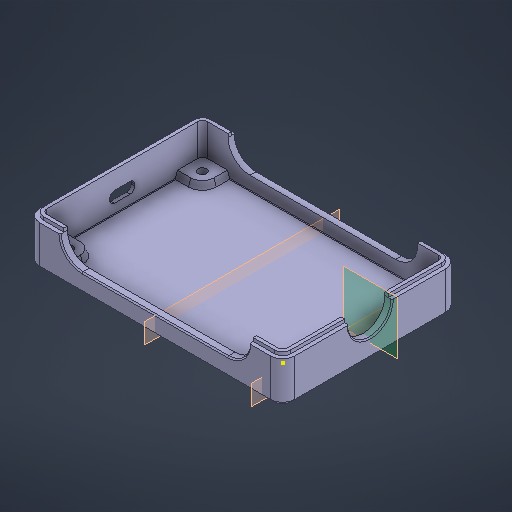
# Autodesk Inventor part: case1
Saved by Autodesk Inventor 2025.2 (Build 292293000, 293)
## iProperties
Created: 2025-10-04
Part Number: case1
Material: Generic
Document SubType Name: Modeling
Designer: micyg
Density: 1 g/cm^3
Appearance: Default
Author: micyg
## iProperties of the stored document case1_3DPrint.ipt
Created: 2025-10-05
Part Number: case1_3DPrint
Material: Generic
Document SubType Name: Modeling
Designer: micyg
Density: 1 g/cm^3
Appearance: Default
Author: micyg
Autodesk Inventor part; units mm, degrees
ref_plane "YZ Plane" through (0, 0, 0) normal (1, 0, 0) x (0, 1, 0)
ref_plane "XZ Plane" through (0, 0, 0) normal (0, 1, 0) x (-1, 0, 0)
ref_plane "XY Plane" through (0, 0, 0) normal (0, 0, 1) x (1, 0, 0)
sketch "Sketch1" plane through (0, 0, 0) normal (0, 1, 0) x (-1, 0, 0)
  line L0 (0, 0) -> (105.2, 0)
  line L1 (105.2, 0) -> (105.2, -72.2)
  line L2 (105.2, -72.2) -> (0, -72.2)
  line L3 (0, -72.2) -> (0, 0)
  line L4 (0, -72.2) -> (105.2, 0) construction
  line L5 (3.6, -3.6) -> (101.6, -3.6) construction
  line L6 (101.6, -3.6) -> (101.6, -68.6) construction
  line L7 (101.6, -68.6) -> (3.6, -68.6) construction
  line L8 (3.6, -68.6) -> (3.6, -3.6) construction
  line L9 (3.6, -3.6) -> (101.6, -68.6) construction
  line L10 (101.6, -3.6) -> (3.6, -68.6) construction
  point P0 (52.6, -36.1)
  dimension "d17" = 98
  dimension "d18" = 65
  dimension "d21" = 72.2
  dimension "d22" = 105.2
  constraints: 22 end point, 4 parallel, 3 midpoint, 2 horizontal, 2 perpendicular
  measures "d17" distance of L6.end L7.end
  measures "d18" distance of L5.end L6.end
  measures "d21" distance between parallel lines of L2 L0
  measures "d22" distance between parallel lines of L3 L1
extrude "Extrusion1" add sketch "Sketch1" along normal blind 17.5
ref_plane "Work Plane7" through (0, 17.5, -36.1) normal (0, 0, -1) x (-1, 0, 0)
fillet "Fillet3" radius 5 4 edges at (-105.2, 8.75, -72.2) (-105.2, 8.75, 0) (0, 8.75, -72.2) (0, 8.75, 0)
chamfer "Chamfer1" distance 2 angle 45 8 edges at (0, 0, -36.1) (-1.4645, 0, -70.7355) (-52.6, 0, -72.2) (-103.7355, 0, -70.7355) (-105.2, 0, -36.1) (-103.7355, 0, -1.4645) (-52.6, 0, 0) (-1.4645, 0, -1.4645)
shell "Shell2" thickness 3 removed faces 1 at (-36.7333, 17.5, -48.1333)
sketch "Sketch2" plane through (-100.2, 3, -69.2) normal (0, 1, 0) x (1, 0, 0)
  line L0 (91.5, -5.6) -> (3.5, -5.6) construction
  line L1 (3.5, -5.6) -> (3.5, -60.6) construction
  line L2 (3.5, -60.6) -> (91.5, -60.6) construction
  line L3 (91.5, -60.6) -> (91.5, -5.6) construction
  arc A0 (91.5, -55.85) -> (86.75, -60.6) centre (91.5, -60.6) ccw
  line L4 (95, 0) -> (0, 0) construction
  arc A1 (-2, -64.2) -> (0, -66.2) centre (0, -64.2) ccw projected
  line L5 (-2, -64.2) -> (-2, -2) projected
  arc A2 (0, 0) -> (-2, -2) centre (0, -2) ccw projected
  line L6 (0, 0) -> (95.2, 0) projected
  arc A3 (97.2, -2) -> (95.2, 0) centre (95.2, -2) ccw projected
  line L7 (97.2, -2) -> (97.2, -64.2) projected
  arc A4 (95.2, -66.2) -> (97.2, -64.2) centre (95.2, -64.2) ccw projected
  line L8 (95.2, -66.2) -> (0, -66.2) projected
  arc A5 (95.2, -69.2) -> (100.2, -64.2) centre (95.2, -64.2) ccw projected
  line L9 (100.2, -64.2) -> (100.2, -2) projected
  arc A6 (100.2, -2) -> (95.2, 3) centre (95.2, -2) ccw projected
  line L10 (95.2, 3) -> (0, 3) projected
  arc A7 (0, 3) -> (-5, -2) centre (0, -2) ccw projected
  line L11 (-5, -2) -> (-5, -64.2) projected
  arc A8 (-5, -64.2) -> (0, -69.2) centre (0, -64.2) ccw projected
  line L12 (0, -69.2) -> (95.2, -69.2) projected
  line L13 (91.5, -55.85) -> (97.2, -55.85)
  line L14 (86.75, -60.6) -> (86.75, -66.2)
  circle A9 centre (91.5, -60.6) radius 1.75
  line L15 (-5, -2) -> (-5, -64.2) projected
  line L16 (-5, -33.1) -> (100.2, -33.1) construction
  line L17 (47.6, -69.2) -> (47.6, 3) construction
  line L18 (3.5, -60.6) -> (91.5, -5.6) construction
  line L19 (47.5, -5.6) -> (47.5, -60.6) construction
  line L20 (-1.5, -0.6) -> (96.5, -0.6) construction
  line L21 (96.5, -0.6) -> (96.5, -65.6) construction
  line L22 (96.5, -65.6) -> (-1.5, -65.6) construction
  line L23 (-1.5, -65.6) -> (-1.5, -0.6) construction
  line L24 (-1.5, -0.6) -> (96.5, -65.6) construction
  arc A10 (86.75, -5.6) -> (91.5, -10.35) centre (91.5, -5.6) ccw
  line L25 (91.5, -10.35) -> (97.2, -10.35)
  line L26 (86.75, -5.6) -> (86.75, 0)
  circle A11 centre (91.5, -5.6) radius 1.75
  arc A12 (8.25, -60.6) -> (3.5, -55.85) centre (3.5, -60.6) ccw
  line L27 (8.25, -60.6) -> (8.25, -66.2)
  circle A13 centre (3.5, -60.6) radius 1.75
  arc A14 (3.5, -10.35) -> (8.25, -5.6) centre (3.5, -5.6) ccw
  line L28 (8.25, -5.6) -> (8.25, 0)
  circle A15 centre (3.5, -5.6) radius 1.75
  line L29 (3.5, -10.35) -> (-2, -10.35)
  line L30 (3.5, -55.85) -> (-2, -55.85)
  point P0 (100.2, -69.2)
  point P1 (47.5, -33.1)
  point P2 (47.5, -33.1)
  point P3 (97.2, -10.35)
  point P4 (8.25, 0)
  dimension "d13" = 88
  dimension "d14" = 55
  dimension "d25" = 3.5
  dimension "d26" = 3
  dimension "d73" = 65
  dimension "d74" = 98
  dimension "d75" = 0.5
  dimension "d76" = 0.7
  constraints: 42 end point, 16 symmetric about line, 9 midpoint, 9 point on circle, 8 centre point, 7 point on line, 4 parallel, 3 coincident, 3 perpendicular, 3 tangent, 2 horizontal, 6 other
  measures "d13" distance between parallel lines of L1 L3
  measures "d14" distance of L2.end L0.start
  measures "d25" diameter of A9
  measures "d26" radial gap between concentric circles of A0 A9
  measures "d73" distance of L20.end L21.end
  measures "d74" distance of L20.start L20.end
  measures "d75" distance between parallel lines of L5 L23
  measures "d76" distance between parallel lines of L21 L7
extrude "Extrusion2" add sketch "Sketch2" along normal blind 2.75 contours L13 L7 A4 L8 L14 A0 | L25 A10 L26 L6 A3 L7 | L8 A1 L5 L30 A12 L27 | L28 A14 L29 L5 A2 L6
ref_plane "Work Plane1" through (-52.6, 17.5, -3) normal (-1, 0, 0) x (0, -1, 0)
ref_plane "Work Plane2" through (-3, 17.5, -36.1) normal (0, 0, 1) x (1, 0, 0)
ref_plane "Work Plane5" through (-52.7, 3, -36.1) normal (1, 0, 0) x (0, 0, -1)
ref_plane "Work Plane6" through (-8.7, 3, -8.6) normal (1, 0, 0) x (0, 0, -1)
sketch "Sketch12" plane through (-8.7, 3, -8.6) normal (1, 0, 0) x (0, 0, -1)
  line L0 (0, 2.75) -> (-5.6, 2.75) projected
  line L1 (-3.6, 2.75) -> (-5.6, 2.75) projected
  line L2 (4.75, 2.75) -> (-3.6, 2.75) projected
  line L3 (4.75, 2.75) -> (0, 2.75) projected
  line L4 (-1.75, 2.75) -> (1.75, 2.75) projected
  line L5 (-1.75, 2.75) -> (1.75, 2.75) projected
  line L6 (1.75, 0) -> (-1.75, 0) projected
  line L7 (-1.75, 2.75) -> (-1.75, 0) projected
  line L8 (1.75, 2.75) -> (1.75, 0) projected
  line L9 (-8.6, 14.5) -> (-8.6, -1) projected
  line L10 (-8.6, -1) -> (-8.6, 14.5) projected
  line L11 (-1.75, 0) -> (-3, -1.25)
  line L12 (-3, -1.25) -> (-3, -3)
  line L13 (-1.75, 0) -> (0, 0)
  line L14 (-1.75, 0) -> (0, 0)
  line L15 (0, 0) -> (0, -3)
  line L16 (1.75, 0) -> (3, -1.25)
  line L17 (3, -1.25) -> (3, -3)
  line L18 (-6.6, -3) -> (-8.6, -1) projected
  line L19 (-8.6, -1) -> (-3.6, -1) projected
  line L20 (-3.6, -3) -> (-3.6, -1) projected
  line L21 (-3.6, -3) -> (-6.6, -3) projected
  line L22 (-3.6, -3) -> (-3.6, -1) projected
  line L23 (-3.6, -1) -> (58.6, -1) projected
  line L24 (58.6, -3) -> (58.6, -1) projected
  line L25 (58.6, -3) -> (-3.6, -3) projected
  line L26 (-8.6, -1) -> (-3.6, -1) projected
  line L27 (-8.6, -1) -> (-8.6, 14.5) projected
  line L28 (-8.6, 14.5) -> (-3.6, 14.5) projected
  line L29 (-3.6, 14.5) -> (-3.6, -1) projected
  point P0 (-8.6, -3)
  dimension "d77" = 45
  dimension "d78" = 6
  constraints: 14 end point, 3 symmetric about line, 2 point on line, 1 collinear, 1 midpoint, 1 perpendicular
  measures "d77" angle of L12 L11
  measures "d78" distance between parallel lines of L17 L12
revolve "Revolution2" cut sketch "Sketch12" angle 360 about axis through (-8.7, 3, -8.6) along (0, -1, 0) contours L16 L23 L15 L6 | L16 L17 L25 L15 L23
mirror "Mirror6" about plane through (-3, 17.5, -36.1) normal (0, 0, 1) of "Revolution2"
mirror "Mirror7" about plane through (-52.7, 3, -36.1) normal (1, 0, 0) of "Revolution2", "Mirror6"
draft "FaceDraft1" angle 20 pull direction (0, 1, 0) faces at (-11.3758, 4.8333, -12.5246) (-13.45, 4.8333, -4.9475) (-4.9809, 4.8333, -13.35) (-13.4367, 3.9167, -63.245) (-4.9809, 4.8333, -58.85) (-13.45, 4.8333, -67.2525) (-92.7754, 4.8333, -11.2758) (-100.2858, 4.8333, -13.35) (-91.95, 4.8333, -4.9475) (-94.9646, 4.8333, -59.1783) (-91.95, 4.8333, -67.2525) (-100.2858, 4.8333, -58.85) fixed edges at (-12.0588, 5.75, -11.9588) (-13.45, 5.75, -5.8) (-5.85, 5.75, -13.35) (-12.0588, 5.75, -60.2412) (-5.85, 5.75, -58.85) (-13.45, 5.75, -66.4) (-93.3412, 5.75, -11.9588) (-99.45, 5.75, -13.35) (-91.95, 5.75, -5.8) (-93.3412, 5.75, -60.2412) (-91.95, 5.75, -66.4) (-99.45, 5.75, -58.85)
sketch "Sketch19" plane through (-5, 17.5, -72.2) normal (0, 0, -1) x (-1, 0, 0)
  line L0 (95.2, -15.5) -> (0, -15.5) construction
  line L1 (95.2, 0) -> (95.2, -15.5) construction
  line L2 (0, 0) -> (95.2, 0) construction
  line L3 (0, -15.5) -> (0, 0) construction
  line L4 (47.7, -21.28) -> (47.7, 5.18) construction
  line L5 (8.7, -9) -> (86.7, -9) construction
  line L6 (86.7, -9) -> (86.7, 9)
  line L7 (86.7, 9) -> (8.7, 9)
  line L8 (8.7, 9) -> (8.7, -9)
  line L9 (8.7, -9) -> (86.7, 9) construction
  line L10 (86.7, -9) -> (8.7, 9) construction
  arc A0 (77.7, -9) -> (77.7, 9) centre (77.7, 0) ccw
  arc A1 (17.7, 9) -> (17.7, -9) centre (17.7, 0) ccw
  line L11 (17.7, -9) -> (77.7, -9)
  line L12 (77.7, 9) -> (17.7, 9)
  point P0 (-5, -17.5)
  point P1 (47.7, 0)
  point P2 (86.7, 0)
  point P3 (8.7, 0)
  point P4 (47.7, 0)
  point P5 (47.7, 0)
  dimension "d103" = 78
  dimension "d104" = 9
  constraints: 16 end point, 8 point on line, 5 tangent, 4 midpoint, 4 point on circle, 2 centre point, 2 horizontal, 2 parallel, 1 perpendicular
  measures "d103" distance between parallel lines of L8 L6
  measures "d104" radius of A0
extrude "Extrusion13" cut sketch "Sketch19" against normal up to surface (3 mm away)
mirror "Mirror9" about plane through (0, 17.5, -36.1) normal (0, 0, -1) of "Extrusion13"
sketch "Sketch20" plane through (0, 17.5, -5) normal (1, 0, 0) x (0, 0, -1)
  line L0 (62.2, -15.5) -> (0, -15.5) construction
  line L1 (62.2, 0) -> (62.2, -15.5) construction
  line L2 (0, 0) -> (62.2, 0) construction
  line L3 (0, -15.5) -> (0, 0) construction
  line L4 (31.1, 3.5) -> (31.1, -21) construction
  circle A0 centre (31.1, 0) radius 9
  point P0 (-5, -17.5)
  dimension "d109" = 18
  constraints: 1 centre point, 1 midpoint, 1 point on line
  measures "d109" diameter of A0
extrude "Extrusion14" cut sketch "Sketch20" against normal up to surface (3 mm away)
sketch "Sketch21" plane through (-105.2, 17.5, -67.2) normal (-1, 0, 0) x (0, 0, 1)
  line L0 (31.1, -9.65) -> (31.1, -9.85) projected
  line L1 (34.29, -9.85) -> (31.1, -9.85) projected
  arc A0 (34.29, -9.85) -> (35.57, -8.57) centre (34.29, -8.57) ccw projected
  line L2 (35.57, -7.97) -> (35.57, -8.57) projected
  arc A1 (35.57, -7.97) -> (34.29, -6.69) centre (34.29, -7.97) ccw projected
  line L3 (31.1, -6.69) -> (34.29, -6.69) projected
  line L4 (31.1, -6.69) -> (31.1, -6.89) projected
  line L5 (31.1, -6.89) -> (34.29, -6.89) projected
  arc A2 (35.37, -7.97) -> (34.29, -6.89) centre (34.29, -7.97) ccw projected
  line L6 (35.37, -7.97) -> (35.37, -8.57) projected
  arc A3 (34.29, -9.65) -> (35.37, -8.57) centre (34.29, -8.57) ccw projected
  line L7 (34.29, -9.65) -> (31.1, -9.65) projected
  line L8 (31.1, -9.65) -> (31.1, -9.85) projected
  line L9 (27.91, -9.65) -> (31.1, -9.65) projected
  arc A4 (26.83, -8.57) -> (27.91, -9.65) centre (27.91, -8.57) ccw projected
  line L10 (26.83, -7.97) -> (26.83, -8.57) projected
  arc A5 (27.91, -6.89) -> (26.83, -7.97) centre (27.91, -7.97) ccw projected
  line L11 (31.1, -6.89) -> (27.91, -6.89) projected
  line L12 (31.1, -6.69) -> (31.1, -6.89) projected
  line L13 (31.1, -6.69) -> (27.91, -6.69) projected
  arc A6 (27.91, -6.69) -> (26.63, -7.97) centre (27.91, -7.97) ccw projected
  line L14 (26.63, -7.97) -> (26.63, -8.57) projected
  arc A7 (26.63, -8.57) -> (27.91, -9.85) centre (27.91, -8.57) ccw projected
  line L15 (27.91, -9.85) -> (31.1, -9.85) projected
  line L16 (31.1, -5.99) -> (34.29, -5.99)
  arc A8 (36.27, -7.97) -> (34.29, -5.99) centre (34.29, -7.97) ccw
  line L17 (36.27, -7.97) -> (36.27, -8.57)
  arc A9 (34.29, -10.55) -> (36.27, -8.57) centre (34.29, -8.57) ccw
  line L18 (34.29, -10.55) -> (31.1, -10.55)
  line L19 (31.1, -5.99) -> (27.91, -5.99)
  arc A10 (27.91, -5.99) -> (25.93, -7.97) centre (27.91, -7.97) ccw
  line L20 (25.93, -7.97) -> (25.93, -8.57)
  arc A11 (25.93, -8.57) -> (27.91, -10.55) centre (27.91, -8.57) ccw
  line L21 (27.91, -10.55) -> (31.1, -10.55)
  point P0 (67.2, -17.5)
  dimension "d112" = 0.7
  constraints: 12 end point, 8 point on circle, 4 centre point, 8 other
  measures "d112" distance between parallel lines of L16 L3
extrude "Extrusion15" cut sketch "Sketch21" against normal up to surface (3 mm away) contours L7 A3 L6 A2 L5 L4 L3 A1 L2 A0 L1 L0 | L9 A4 L10 A5 L11 L5 A2 L6 A3 L7 | L0 L15 A7 L14 A6 L13 L4 L11 A5 L10 A4 L9 | L16 A8 L17 A9 L18 L21 A11 L20 A10 L19
sketch "Sketch22" plane through (0, 17.5, -36.1) normal (0, 0, -1) x (-1, 0, 0)
  line L0 (102.2, -5.99) -> (102.2, -7.97) projected
  line L1 (105.2, -5.99) -> (102.2, -5.99) projected
  line L2 (105.2, -7.97) -> (105.2, -5.99) projected
  line L3 (105.2, -7.97) -> (102.2, -7.97) projected
  line L4 (102.2, -8.57) -> (102.2, -10.55) projected
  line L5 (105.2, -8.57) -> (102.2, -8.57) projected
  line L6 (105.2, -10.55) -> (105.2, -8.57) projected
  line L7 (105.2, -10.55) -> (102.2, -10.55) projected
  line L8 (102.2, -7.97) -> (102.2, -8.57) projected
  line L9 (105.2, -7.97) -> (102.2, -7.97) projected
  line L10 (105.2, -8.57) -> (105.2, -7.97) projected
  line L11 (105.2, -8.57) -> (102.2, -8.57) projected
  line L12 (105.2, -5.99) -> (102.2, -5.99) projected
  line L13 (105.2, -5.99) -> (102.2, -5.99) projected
  line L14 (105.2, -10.55) -> (102.2, -10.55) projected
  line L15 (105.2, -10.55) -> (102.2, -10.55) projected
  line L16 (105.2, -5.99) -> (105.2, -7.97) projected
  line L17 (105.2, -7.97) -> (105.2, -8.57) projected
  line L18 (105.2, -8.57) -> (105.2, -10.55) projected
  line L19 (105.2, -10.55) -> (105.2, -8.57) projected
  line L20 (105.2, -8.57) -> (105.2, -7.97) projected
  line L21 (105.2, -7.97) -> (105.2, -5.99) projected
  line L22 (105.2, 0) -> (105.2, -15.5) projected
  line L23 (105.2, -15.5) -> (105.2, 0) projected
  line L24 (103.7, -10.55) -> (103.7, -11.85)
  line L25 (103.7, -11.85) -> (105.2, -13.1086)
  point P0 (0, -17.5)
  point P1 (103.7, -10.55)
  dimension "d116" = 50
  dimension "d123" = 1.3
  constraints: 4 end point, 1 midpoint, 1 point on line, 1 vertical
  measures "d116" angle of L24 L25
  measures "d123" distance from line of L7 L24.end
sketch3d "3D Sketch3"
  line L0 (-105.2, 6.95, -39.29) -> (-105.2, 6.95, -32.91)
  arc A0 (-105.2, 6.95, -32.91) -> (-105.2, 8.93, -30.93) centre (-105.2, 8.93, -32.91) ccw
  line L1 (-105.2, 8.93, -30.93) -> (-105.2, 9.53, -30.93)
  arc A1 (-105.2, 9.53, -30.93) -> (-105.2, 11.51, -32.91) centre (-105.2, 9.53, -32.91) ccw
  line L2 (-105.2, 11.51, -32.91) -> (-105.2, 11.51, -39.29)
  arc A2 (-105.2, 11.51, -39.29) -> (-105.2, 9.53, -41.27) centre (-105.2, 9.53, -39.29) ccw
  line L3 (-105.2, 9.53, -41.27) -> (-105.2, 8.93, -41.27)
  arc A3 (-105.2, 8.93, -41.27) -> (-105.2, 6.95, -39.29) centre (-105.2, 8.93, -39.29) ccw
sweep "Sweep2" cut profiles "Sketch22" path "3D Sketch3" contours L22 L25 L24 L7
sketch "Sketch23" plane through (0, 17.5, 0) normal (0, 1, 0) x (1, 0, 0)
  point P0 (0, 0)
sketch "Sketch24" plane through (0, 17.5, 0) normal (0, 1, 0) x (1, 0, 0)
  line L0 (-91.7, 0) -> (-91.7, 3) projected
  line L1 (-91.7, 3) -> (-100.2, 3) projected
  arc A0 (-102.2, 5) -> (-100.2, 3) centre (-100.2, 5) ccw projected
  line L2 (-102.2, 5) -> (-102.2, 67.2) projected
  arc A1 (-100.2, 69.2) -> (-102.2, 67.2) centre (-100.2, 67.2) ccw projected
  line L3 (-100.2, 69.2) -> (-91.7, 69.2) projected
  line L4 (-91.7, 69.2) -> (-91.7, 72.2) projected
  line L5 (-91.7, 72.2) -> (-100.2, 72.2) projected
  arc A2 (-100.2, 72.2) -> (-105.2, 67.2) centre (-100.2, 67.2) ccw projected
  line L6 (-105.2, 67.2) -> (-105.2, 5) projected
  arc A3 (-105.2, 5) -> (-100.2, 0) centre (-100.2, 5) ccw projected
  line L7 (-100.2, 0) -> (-91.7, 0) projected
  line L8 (-3, 45.1) -> (0, 45.1) projected
  line L9 (0, 45.1) -> (0, 67.2) projected
  arc A4 (0, 67.2) -> (-5, 72.2) centre (-5, 67.2) ccw projected
  line L10 (-5, 72.2) -> (-13.7, 72.2) projected
  line L11 (-13.7, 72.2) -> (-13.7, 69.2) projected
  line L12 (-13.7, 69.2) -> (-5, 69.2) projected
  arc A5 (-3, 67.2) -> (-5, 69.2) centre (-5, 67.2) ccw projected
  line L13 (-3, 67.2) -> (-3, 45.1) projected
  line L14 (0, 27.1) -> (-3, 27.1) projected
  line L15 (-3, 27.1) -> (-3, 5) projected
  arc A6 (-5, 3) -> (-3, 5) centre (-5, 5) ccw projected
  line L16 (-5, 3) -> (-13.7, 3) projected
  line L17 (-13.7, 3) -> (-13.7, 0) projected
  line L18 (-13.7, 0) -> (-5, 0) projected
  arc A7 (-5, 0) -> (0, 5) centre (-5, 5) ccw projected
  line L19 (0, 5) -> (0, 27.1) projected
  line L20 (-3, 45.1) -> (0, 45.1) projected
  line L21 (-3, 27.1) -> (-3, 45.1) projected
  line L22 (0, 27.1) -> (-3, 27.1) projected
  line L23 (0, 45.1) -> (0, 27.1) projected
  line L24 (-13.7, 72.2) -> (-13.7, 69.2) projected
  line L25 (-1.6, 67.2) -> (-1.6, 5)
  line L26 (0, 5) -> (0, 27.1) projected
  arc A8 (-5, 1.6) -> (-1.6, 5) centre (-5, 5) ccw
  arc A9 (-5, 3) -> (-3, 5) centre (-5, 5) ccw projected
  line L27 (-13.7, 1.6) -> (-5, 1.6)
  arc A10 (-1.6, 67.2) -> (-5, 70.6) centre (-5, 67.2) ccw
  line L28 (-5, 70.6) -> (-13.7, 70.6)
  arc A11 (-3, 67.2) -> (-5, 69.2) centre (-5, 67.2) ccw projected
  line L29 (-91.7, 69.2) -> (-91.7, 72.2) projected
  line L30 (-91.7, 70.6) -> (-100.2, 70.6)
  line L31 (-103.6, 67.2) -> (-103.6, 5)
  line L32 (-100.2, 1.6) -> (-91.7, 1.6)
  arc A12 (-103.6, 5) -> (-100.2, 1.6) centre (-100.2, 5) ccw
  arc A13 (-100.2, 70.6) -> (-103.6, 67.2) centre (-100.2, 67.2) ccw
  point P0 (0, 0)
  point P1 (-1.6, 27.1)
  point P2 (-1.6, 45.1)
  dimension "d119" = 1.4
  dimension "d120" = 1.4
  constraints: 12 end point, 8 point on circle, 8 tangent, 6 parallel, 4 centre point, 4 concentric, 4 point on line
  measures "d119" distance between parallel lines of L15 L25
  measures "d120" distance between parallel lines of L1 L32
extrude "Extrusion16" add sketch "Sketch24" along normal blind 1.4 contours L32 A12 L31 A13 L30 L4 L3 A1 L2 A0 L1 L0 | L13 A5 L12 L11 L28 A10 L25 L8 | L14 L25 A8 L27 L17 L16 A6 L15
chamfer "Chamfer2" distance 0.5 angle 45 7 edges at (-16.336, 11.136, -72.2) (-52.7, 8.5, -72.2) (-89.064, 11.136, -72.2) (-89.064, 11.136, 0) (-52.7, 8.5, 0) (-16.336, 11.136, 0) (0, 8.5, -36.1)
body "Solid1"
